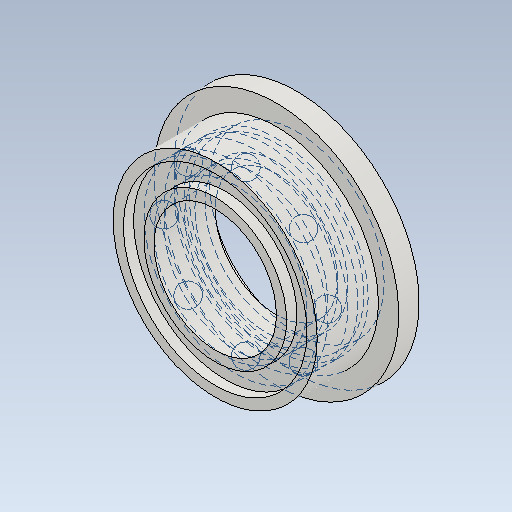
# Autodesk Inventor part: φ6φ10ベアリング
Saved by Autodesk Inventor 2020 (Build 240168000, 168)
## iProperties
Created: 2020-02-02
Part Number: φ6φ10ベアリング
Material: 鋼 AISI 1006 85 HR
Document SubType Name: Modeling
Designer: happy
Density: 7.872 g/cm^3
Appearance: 鋼
Mass: 1.26042 g
Surface Area: 5.72828 cm^2
Volume: 0.160114 cm^3
Author: happy
Autodesk Inventor part; units mm, degrees
ref_plane "YZ Plane" through (0, 0, 0) normal (1, 0, 0) x (0, 1, 0)
ref_plane "XZ Plane" through (0, 0, 0) normal (0, 1, 0) x (-1, 0, 0)
ref_plane "XY Plane" through (0, 0, 0) normal (0, 0, 1) x (1, 0, 0)
sketch "スケッチ1" plane through (0, 0, 0) normal (0, 0, 1) x (1, 0, 0)
  circle A0 centre (0, 0) radius 3
  circle A1 centre (0, 0) radius 3.5
  circle A2 centre (0, 0) radius 5
  circle A3 centre (0, 0) radius 4.5
  dimension "d0" = 6
  dimension "d1" = 7
  dimension "d2" = 10
  dimension "d3" = 9
  constraints: 4 centre point, 4 coincident
  measures "d0" diameter of A0
  measures "d1" diameter of A1
  measures "d2" diameter of A2
  measures "d3" diameter of A3
extrude "押し出し1" add sketch "スケッチ1" along normal blind 3
sketch "スケッチ2" plane through (0, 0, 3) normal (0, 0, 1) x (1, 0, 0)
  point P0 (0, 0)
ref_plane "作業平面1" through (0, 0, 2) normal (0, 0, 1) x (1, 0, 0)
ref_plane "作業平面2" through (0, 0, 1) normal (0, 0, -1) x (-1, 0, 0)
ref_plane "作業平面3" through (0, 0, 1.5) normal (0, 0, -1) x (-1, 0, 0)
sketch "スケッチ3" plane through (0, 0, 1.5) normal (0, 0, -1) x (-1, 0, 0)
  circle A0 centre (0, 4) radius 0.5
  circle A1 centre (0, 0) radius 4.5 projected
  circle A2 centre (0, 0) radius 3.5 projected
  line L0 (0, 4.5) -> (0, 3.5)
  constraints: 2 end point, 2 point on circle, 2 vertical alignment, 1 centre point, 4 other
revolve "回転1" add sketch "スケッチ3" angle 360 about axis through (0, 4.5, 1.5) along (0, -1, 0) picked at (0.0723, 4.1502) contours A0 L0
pattern_circular "円形状パターン1" count 8 over 360 about axis through (0, 0, -10) along (0, 0, 1) of "回転1"
sketch "スケッチ4" plane through (0, 0, 1) normal (0, 0, -1) x (-1, 0, 0)
  circle A0 centre (0, 0) radius 3.5 projected
  circle A1 centre (0, 0) radius 4.5 projected
extrude "押し出し2" add sketch "スケッチ4" along normal blind 0.5
sketch "スケッチ5" plane through (0, 0, 2) normal (0, 0, 1) x (1, 0, 0)
  circle A0 centre (0, 0) radius 3.5 projected
  circle A1 centre (0, 0) radius 4.5 projected
extrude "押し出し3" add sketch "スケッチ5" along normal blind 0.5
sketch "スケッチ6" plane through (0, 0, 0) normal (0, 0, -1) x (-1, 0, 0)
  circle A0 centre (0, 0) radius 4.2857
  circle A1 centre (0, 0) radius 6
  dimension "d17" = 12
  constraints: 2 centre point, 2 coincident
  measures "d17" diameter of A1
extrude "押し出し4" add sketch "スケッチ6" along normal blind 1
sketch "スケッチ7" plane through (0, 0, 0) normal (0, 0, -1) x (-1, 0, 0)
  point P0 (0, 0)
